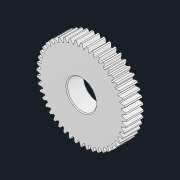
# Autodesk Inventor part: unit-planet_gear
Saved by Autodesk Inventor 2021 (Build 250183000, 183)
## iProperties
Created: 2021-07-12
Part Number: unit-planet_gear
Material: ABS プラスチック
Document SubType Name: Modeling
Designer: yuta0
Density: 1.06 g/cm^3
Appearance: 滑らか - 白
購入先: 印刷
在庫数: 0.0
Author: yuta0
Autodesk Inventor part; units mm, degrees
ref_plane "YZ Plane" through (0, 0, 0) normal (1, 0, 0) x (0, 1, 0)
ref_plane "XZ Plane" through (0, 0, 0) normal (0, 1, 0) x (-1, 0, 0)
ref_plane "XY Plane" through (0, 0, 0) normal (0, 0, 1) x (1, 0, 0)
sketch "スケッチ1" plane through (0, 0, 0) normal (0, 0, 1) x (1, 0, 0)
  arc A0 (-3.6816, 24.8194) -> (-4.0891, 22.473) centre (7.7013, 21.6341) ccw
  arc A1 (-4.0891, 22.473) -> (-4.8222, 22.3272) centre (0, 0) ccw
  arc A2 (-4.8222, 22.3272) -> (-6.0966, 24.3391) centre (-15.394, 17.0401) ccw
  arc A3 (-6.0966, 24.3391) -> (-6.8897, 24.1266) centre (0, 0) ccw
  arc A4 (-6.8897, 24.1266) -> (-6.9874, 21.747) centre (4.8116, 22.4542) ccw
  arc A5 (-6.9874, 21.747) -> (-7.6952, 21.5067) centre (0, 0) ccw
  arc A6 (-7.6952, 21.5067) -> (-9.2213, 23.3351) centre (-17.4865, 14.885) ccw
  arc A7 (-9.2213, 23.3351) -> (-9.9799, 23.0209) centre (0, 0) ccw
  arc A8 (-9.9799, 23.0209) -> (-9.7662, 20.6489) centre (1.8395, 22.8902) ccw
  arc A9 (-9.7662, 20.6489) -> (-10.4366, 20.3183) centre (0, 0) ccw
  arc A10 (-10.4366, 20.3183) -> (-12.1883, 21.9318) centre (-19.2798, 12.4752) ccw
  arc A11 (-12.1883, 21.9318) -> (-12.8994, 21.5213) centre (0, 0) ccw
  arc A12 (-12.8994, 21.5213) -> (-12.3779, 19.1975) centre (-1.164, 22.9344) ccw
  arc A13 (-12.3779, 19.1975) -> (-12.9994, 18.7822) centre (0, 0) ccw
  arc A14 (-12.9994, 18.7822) -> (-14.9467, 20.1533) centre (-20.7432, 9.852) ccw
  arc A15 (-14.9467, 20.1533) -> (-15.5981, 19.6535) centre (0, 0) ccw
  arc A16 (-15.5981, 19.6535) -> (-14.7778, 17.4176) centre (-4.1476, 22.5863) ccw
  arc A17 (-14.7778, 17.4176) -> (-15.3397, 16.9248) centre (0, 0) ccw
  arc A18 (-15.3397, 16.9248) -> (-17.4494, 18.0299) centre (-21.8517, 7.0602) ccw
  arc A19 (-17.4494, 18.0299) -> (-18.0299, 17.4494) centre (0, 0) ccw
  arc A20 (-18.0299, 17.4494) -> (-16.9248, 15.3397) centre (-7.0602, 21.8517) ccw
  arc A21 (-16.9248, 15.3397) -> (-17.4176, 14.7778) centre (0, 0) ccw
  arc A22 (-17.4176, 14.7778) -> (-19.6535, 15.5981) centre (-22.5863, 4.1476) ccw
  arc A23 (-19.6535, 15.5981) -> (-20.1533, 14.9467) centre (0, 0) ccw
  arc A24 (-20.1533, 14.9467) -> (-18.7822, 12.9994) centre (-9.852, 20.7432) ccw
  arc A25 (-18.7822, 12.9994) -> (-19.1975, 12.3779) centre (0, 0) ccw
  arc A26 (-19.1975, 12.3779) -> (-21.5213, 12.8994) centre (-22.9344, 1.164) ccw
  arc A27 (-21.5213, 12.8994) -> (-21.9318, 12.1883) centre (0, 0) ccw
  arc A28 (-21.9318, 12.1883) -> (-20.3183, 10.4366) centre (-12.4752, 19.2798) ccw
  arc A29 (-20.3183, 10.4366) -> (-20.6489, 9.7662) centre (0, 0) ccw
  arc A30 (-20.6489, 9.7662) -> (-23.0209, 9.9799) centre (-22.8902, -1.8395) ccw
  arc A31 (-23.0209, 9.9799) -> (-23.3351, 9.2213) centre (0, 0) ccw
  arc A32 (-23.3351, 9.2213) -> (-21.5067, 7.6952) centre (-14.885, 17.4865) ccw
  arc A33 (-21.5067, 7.6952) -> (-21.747, 6.9874) centre (0, 0) ccw
  arc A34 (-21.747, 6.9874) -> (-24.1266, 6.8897) centre (-22.4542, -4.8116) ccw
  arc A35 (-24.1266, 6.8897) -> (-24.3391, 6.0966) centre (0, 0) ccw
  arc A36 (-24.3391, 6.0966) -> (-22.3272, 4.8222) centre (-17.0401, 15.394) ccw
  arc A37 (-22.3272, 4.8222) -> (-22.473, 4.0891) centre (0, 0) ccw
  arc A38 (-22.473, 4.0891) -> (-24.8194, 3.6816) centre (-21.6341, -7.7013) ccw
  arc A39 (-24.8194, 3.6816) -> (-24.9266, 2.8676) centre (0, 0) ccw
  arc A40 (-24.9266, 2.8676) -> (-22.7656, 1.8667) centre (-18.9037, 13.0382) ccw
  arc A41 (-22.7656, 1.8667) -> (-22.8145, 1.1208) centre (0, 0) ccw
  arc A42 (-22.8145, 1.1208) -> (-25.0876, 0.4105) centre (-20.4438, -10.4592) ccw
  arc A43 (-25.0876, 0.4105) -> (-25.0876, -0.4105) centre (0, 0) ccw
  arc A44 (-25.0876, -0.4105) -> (-22.8145, -1.1208) centre (-20.4438, 10.4592) ccw
  arc A45 (-22.8145, -1.1208) -> (-22.7656, -1.8667) centre (0, 0) ccw
  arc A46 (-22.7656, -1.8667) -> (-24.9266, -2.8676) centre (-18.9037, -13.0382) ccw
  arc A47 (-24.9266, -2.8676) -> (-24.8194, -3.6816) centre (0, 0) ccw
  arc A48 (-24.8194, -3.6816) -> (-22.473, -4.0891) centre (-21.6341, 7.7013) ccw
  arc A49 (-22.473, -4.0891) -> (-22.3272, -4.8222) centre (0, 0) ccw
  arc A50 (-22.3272, -4.8222) -> (-24.3391, -6.0966) centre (-17.0401, -15.394) ccw
  arc A51 (-24.3391, -6.0966) -> (-24.1266, -6.8897) centre (0, 0) ccw
  arc A52 (-24.1266, -6.8897) -> (-21.747, -6.9874) centre (-22.4542, 4.8116) ccw
  arc A53 (-21.747, -6.9874) -> (-21.5067, -7.6952) centre (0, 0) ccw
  arc A54 (-21.5067, -7.6952) -> (-23.3351, -9.2213) centre (-14.885, -17.4865) ccw
  arc A55 (-23.3351, -9.2213) -> (-23.0209, -9.9799) centre (0, 0) ccw
  arc A56 (-23.0209, -9.9799) -> (-20.6489, -9.7662) centre (-22.8902, 1.8395) ccw
  arc A57 (-20.6489, -9.7662) -> (-20.3183, -10.4366) centre (0, 0) ccw
  arc A58 (-20.3183, -10.4366) -> (-21.9318, -12.1883) centre (-12.4752, -19.2798) ccw
  arc A59 (-21.9318, -12.1883) -> (-21.5213, -12.8994) centre (0, 0) ccw
  arc A60 (-21.5213, -12.8994) -> (-19.1975, -12.3779) centre (-22.9344, -1.164) ccw
  arc A61 (-19.1975, -12.3779) -> (-18.7822, -12.9994) centre (0, 0) ccw
  arc A62 (-18.7822, -12.9994) -> (-20.1533, -14.9467) centre (-9.852, -20.7432) ccw
  arc A63 (-20.1533, -14.9467) -> (-19.6535, -15.5981) centre (0, 0) ccw
  arc A64 (-19.6535, -15.5981) -> (-17.4176, -14.7778) centre (-22.5863, -4.1476) ccw
  arc A65 (-17.4176, -14.7778) -> (-16.9248, -15.3397) centre (0, 0) ccw
  arc A66 (-16.9248, -15.3397) -> (-18.0299, -17.4494) centre (-7.0602, -21.8517) ccw
  arc A67 (-18.0299, -17.4494) -> (-17.4494, -18.0299) centre (0, 0) ccw
  arc A68 (-17.4494, -18.0299) -> (-15.3397, -16.9248) centre (-21.8517, -7.0602) ccw
  arc A69 (-15.3397, -16.9248) -> (-14.7778, -17.4176) centre (0, 0) ccw
  arc A70 (-14.7778, -17.4176) -> (-15.5981, -19.6535) centre (-4.1476, -22.5863) ccw
  arc A71 (-15.5981, -19.6535) -> (-14.9467, -20.1533) centre (0, 0) ccw
  arc A72 (-14.9467, -20.1533) -> (-12.9994, -18.7822) centre (-20.7432, -9.852) ccw
  arc A73 (-12.9994, -18.7822) -> (-12.3779, -19.1975) centre (0, 0) ccw
  arc A74 (-12.3779, -19.1975) -> (-12.8994, -21.5213) centre (-1.164, -22.9344) ccw
  arc A75 (-12.8994, -21.5213) -> (-12.1883, -21.9318) centre (0, 0) ccw
  arc A76 (-12.1883, -21.9318) -> (-10.4366, -20.3183) centre (-19.2798, -12.4752) ccw
  arc A77 (-10.4366, -20.3183) -> (-9.7662, -20.6489) centre (0, 0) ccw
  arc A78 (-9.7662, -20.6489) -> (-9.9799, -23.0209) centre (1.8395, -22.8902) ccw
  arc A79 (-9.9799, -23.0209) -> (-9.2213, -23.3351) centre (0, 0) ccw
  arc A80 (-9.2213, -23.3351) -> (-7.6952, -21.5067) centre (-17.4865, -14.885) ccw
  arc A81 (-7.6952, -21.5067) -> (-6.9874, -21.747) centre (0, 0) ccw
  arc A82 (-6.9874, -21.747) -> (-6.8897, -24.1266) centre (4.8116, -22.4542) ccw
  arc A83 (-6.8897, -24.1266) -> (-6.0966, -24.3391) centre (0, 0) ccw
  arc A84 (-6.0966, -24.3391) -> (-4.8222, -22.3272) centre (-15.394, -17.0401) ccw
  arc A85 (-4.8222, -22.3272) -> (-4.0891, -22.473) centre (0, 0) ccw
  arc A86 (-4.0891, -22.473) -> (-3.6816, -24.8194) centre (7.7013, -21.6341) ccw
  arc A87 (-3.6816, -24.8194) -> (-2.8676, -24.9266) centre (0, 0) ccw
  arc A88 (-2.8676, -24.9266) -> (-1.8667, -22.7656) centre (-13.0382, -18.9037) ccw
  arc A89 (-1.8667, -22.7656) -> (-1.1208, -22.8145) centre (0, 0) ccw
  arc A90 (-1.1208, -22.8145) -> (-0.4105, -25.0876) centre (10.4592, -20.4438) ccw
  arc A91 (-0.4105, -25.0876) -> (0.4105, -25.0876) centre (0, 0) ccw
  arc A92 (0.4105, -25.0876) -> (1.1208, -22.8145) centre (-10.4592, -20.4438) ccw
  arc A93 (1.1208, -22.8145) -> (1.8667, -22.7656) centre (0, 0) ccw
  arc A94 (1.8667, -22.7656) -> (2.8676, -24.9266) centre (13.0382, -18.9037) ccw
  arc A95 (2.8676, -24.9266) -> (3.6816, -24.8194) centre (0, 0) ccw
  arc A96 (3.6816, -24.8194) -> (4.0891, -22.473) centre (-7.7013, -21.6341) ccw
  arc A97 (4.0891, -22.473) -> (4.8222, -22.3272) centre (0, 0) ccw
  arc A98 (4.8222, -22.3272) -> (6.0966, -24.3391) centre (15.394, -17.0401) ccw
  arc A99 (6.0966, -24.3391) -> (6.8897, -24.1266) centre (0, 0) ccw
  arc A100 (6.8897, -24.1266) -> (6.9874, -21.747) centre (-4.8116, -22.4542) ccw
  arc A101 (6.9874, -21.747) -> (7.6952, -21.5067) centre (0, 0) ccw
  arc A102 (7.6952, -21.5067) -> (9.2213, -23.3351) centre (17.4865, -14.885) ccw
  arc A103 (9.2213, -23.3351) -> (9.9799, -23.0209) centre (0, 0) ccw
  arc A104 (9.9799, -23.0209) -> (9.7662, -20.6489) centre (-1.8395, -22.8902) ccw
  arc A105 (9.7662, -20.6489) -> (10.4366, -20.3183) centre (0, 0) ccw
  arc A106 (10.4366, -20.3183) -> (12.1883, -21.9318) centre (19.2798, -12.4752) ccw
  arc A107 (12.1883, -21.9318) -> (12.8994, -21.5213) centre (0, 0) ccw
  arc A108 (12.8994, -21.5213) -> (12.3779, -19.1975) centre (1.164, -22.9344) ccw
  arc A109 (12.3779, -19.1975) -> (12.9994, -18.7822) centre (0, 0) ccw
  arc A110 (12.9994, -18.7822) -> (14.9467, -20.1533) centre (20.7432, -9.852) ccw
  arc A111 (14.9467, -20.1533) -> (15.5981, -19.6535) centre (0, 0) ccw
  arc A112 (15.5981, -19.6535) -> (14.7778, -17.4176) centre (4.1476, -22.5863) ccw
  arc A113 (14.7778, -17.4176) -> (15.3397, -16.9248) centre (0, 0) ccw
  arc A114 (15.3397, -16.9248) -> (17.4494, -18.0299) centre (21.8517, -7.0602) ccw
  arc A115 (17.4494, -18.0299) -> (18.0299, -17.4494) centre (0, 0) ccw
  arc A116 (18.0299, -17.4494) -> (16.9248, -15.3397) centre (7.0602, -21.8517) ccw
  arc A117 (16.9248, -15.3397) -> (17.4176, -14.7778) centre (0, 0) ccw
  arc A118 (17.4176, -14.7778) -> (19.6535, -15.5981) centre (22.5863, -4.1476) ccw
  arc A119 (19.6535, -15.5981) -> (20.1533, -14.9467) centre (0, 0) ccw
  arc A120 (20.1533, -14.9467) -> (18.7822, -12.9994) centre (9.852, -20.7432) ccw
  arc A121 (18.7822, -12.9994) -> (19.1975, -12.3779) centre (0, 0) ccw
  arc A122 (19.1975, -12.3779) -> (21.5213, -12.8994) centre (22.9344, -1.164) ccw
  arc A123 (21.5213, -12.8994) -> (21.9318, -12.1883) centre (0, 0) ccw
  arc A124 (21.9318, -12.1883) -> (20.3183, -10.4366) centre (12.4752, -19.2798) ccw
  arc A125 (20.3183, -10.4366) -> (20.6489, -9.7662) centre (0, 0) ccw
  arc A126 (20.6489, -9.7662) -> (23.0209, -9.9799) centre (22.8902, 1.8395) ccw
  arc A127 (23.0209, -9.9799) -> (23.3351, -9.2213) centre (0, 0) ccw
  arc A128 (23.3351, -9.2213) -> (21.5067, -7.6952) centre (14.885, -17.4865) ccw
  arc A129 (21.5067, -7.6952) -> (21.747, -6.9874) centre (0, 0) ccw
  arc A130 (21.747, -6.9874) -> (24.1266, -6.8897) centre (22.4542, 4.8116) ccw
  arc A131 (24.1266, -6.8897) -> (24.3391, -6.0966) centre (0, 0) ccw
  arc A132 (24.3391, -6.0966) -> (22.3272, -4.8222) centre (17.0401, -15.394) ccw
  arc A133 (22.3272, -4.8222) -> (22.473, -4.0891) centre (0, 0) ccw
  arc A134 (22.473, -4.0891) -> (24.8194, -3.6816) centre (21.6341, 7.7013) ccw
  arc A135 (24.8194, -3.6816) -> (24.9266, -2.8676) centre (0, 0) ccw
  arc A136 (24.9266, -2.8676) -> (22.7656, -1.8667) centre (18.9037, -13.0382) ccw
  arc A137 (22.7656, -1.8667) -> (22.8145, -1.1208) centre (0, 0) ccw
  arc A138 (22.8145, -1.1208) -> (25.0876, -0.4105) centre (20.4438, 10.4592) ccw
  arc A139 (25.0876, -0.4105) -> (25.0876, 0.4105) centre (0, 0) ccw
  arc A140 (25.0876, 0.4105) -> (22.8145, 1.1208) centre (20.4438, -10.4592) ccw
  arc A141 (22.8145, 1.1208) -> (22.7656, 1.8667) centre (0, 0) ccw
  arc A142 (22.7656, 1.8667) -> (24.9266, 2.8676) centre (18.9037, 13.0382) ccw
  arc A143 (24.9266, 2.8676) -> (24.8194, 3.6816) centre (0, 0) ccw
  arc A144 (24.8194, 3.6816) -> (22.473, 4.0891) centre (21.6341, -7.7013) ccw
  arc A145 (22.473, 4.0891) -> (22.3272, 4.8222) centre (0, 0) ccw
  arc A146 (22.3272, 4.8222) -> (24.3391, 6.0966) centre (17.0401, 15.394) ccw
  arc A147 (24.3391, 6.0966) -> (24.1266, 6.8897) centre (0, 0) ccw
  arc A148 (24.1266, 6.8897) -> (21.747, 6.9874) centre (22.4542, -4.8116) ccw
  arc A149 (21.747, 6.9874) -> (21.5067, 7.6952) centre (0, 0) ccw
  arc A150 (21.5067, 7.6952) -> (23.3351, 9.2213) centre (14.885, 17.4865) ccw
  arc A151 (23.3351, 9.2213) -> (23.0209, 9.9799) centre (0, 0) ccw
  arc A152 (23.0209, 9.9799) -> (20.6489, 9.7662) centre (22.8902, -1.8395) ccw
  arc A153 (20.6489, 9.7662) -> (20.3183, 10.4366) centre (0, 0) ccw
  arc A154 (20.3183, 10.4366) -> (21.9318, 12.1883) centre (12.4752, 19.2798) ccw
  arc A155 (21.9318, 12.1883) -> (21.5213, 12.8994) centre (0, 0) ccw
  arc A156 (21.5213, 12.8994) -> (19.1975, 12.3779) centre (22.9344, 1.164) ccw
  arc A157 (19.1975, 12.3779) -> (18.7822, 12.9994) centre (0, 0) ccw
  arc A158 (18.7822, 12.9994) -> (20.1533, 14.9467) centre (9.852, 20.7432) ccw
  arc A159 (20.1533, 14.9467) -> (19.6535, 15.5981) centre (0, 0) ccw
  arc A160 (19.6535, 15.5981) -> (17.4176, 14.7778) centre (22.5863, 4.1476) ccw
  arc A161 (17.4176, 14.7778) -> (16.9248, 15.3397) centre (0, 0) ccw
  arc A162 (16.9248, 15.3397) -> (18.0299, 17.4494) centre (7.0602, 21.8517) ccw
  arc A163 (18.0299, 17.4494) -> (17.4494, 18.0299) centre (0, 0) ccw
  arc A164 (17.4494, 18.0299) -> (15.3397, 16.9248) centre (21.8517, 7.0602) ccw
  arc A165 (15.3397, 16.9248) -> (14.7778, 17.4176) centre (0, 0) ccw
  arc A166 (14.7778, 17.4176) -> (15.5981, 19.6535) centre (4.1476, 22.5863) ccw
  arc A167 (15.5981, 19.6535) -> (14.9467, 20.1533) centre (0, 0) ccw
  arc A168 (14.9467, 20.1533) -> (12.9994, 18.7822) centre (20.7432, 9.852) ccw
  arc A169 (12.9994, 18.7822) -> (12.3779, 19.1975) centre (0, 0) ccw
  arc A170 (12.3779, 19.1975) -> (12.8994, 21.5213) centre (1.164, 22.9344) ccw
  arc A171 (12.8994, 21.5213) -> (12.1883, 21.9318) centre (0, 0) ccw
  arc A172 (12.1883, 21.9318) -> (10.4366, 20.3183) centre (19.2798, 12.4752) ccw
  arc A173 (10.4366, 20.3183) -> (9.7662, 20.6489) centre (0, 0) ccw
  arc A174 (9.7662, 20.6489) -> (9.9799, 23.0209) centre (-1.8395, 22.8902) ccw
  arc A175 (9.9799, 23.0209) -> (9.2213, 23.3351) centre (0, 0) ccw
  arc A176 (9.2213, 23.3351) -> (7.6952, 21.5067) centre (17.4865, 14.885) ccw
  arc A177 (7.6952, 21.5067) -> (6.9874, 21.747) centre (0, 0) ccw
  arc A178 (6.9874, 21.747) -> (6.8897, 24.1266) centre (-4.8116, 22.4542) ccw
  arc A179 (6.8897, 24.1266) -> (6.0966, 24.3391) centre (0, 0) ccw
  arc A180 (6.0966, 24.3391) -> (4.8222, 22.3272) centre (15.394, 17.0401) ccw
  arc A181 (4.8222, 22.3272) -> (4.0891, 22.473) centre (0, 0) ccw
  arc A182 (4.0891, 22.473) -> (3.6816, 24.8194) centre (-7.7013, 21.6341) ccw
  arc A183 (3.6816, 24.8194) -> (2.8676, 24.9266) centre (0, 0) ccw
  arc A184 (2.8676, 24.9266) -> (1.8667, 22.7656) centre (13.0382, 18.9037) ccw
  arc A185 (1.8667, 22.7656) -> (1.1208, 22.8145) centre (0, 0) ccw
  arc A186 (1.1208, 22.8145) -> (0.4105, 25.0876) centre (-10.4592, 20.4438) ccw
  arc A187 (0.4105, 25.0876) -> (-0.4105, 25.0876) centre (0, 0) ccw
  arc A188 (-0.4105, 25.0876) -> (-1.1208, 22.8145) centre (10.4592, 20.4438) ccw
  arc A189 (-1.1208, 22.8145) -> (-1.8667, 22.7656) centre (0, 0) ccw
  arc A190 (-1.8667, 22.7656) -> (-2.8676, 24.9266) centre (-13.0382, 18.9037) ccw
  arc A191 (-2.8676, 24.9266) -> (-3.6816, 24.8194) centre (0, 0) ccw
  constraints: 384 point on circle, 192 centre point, 578 other
extrude "押し出し1" add sketch "スケッチ1" along normal mid plane 9.8
sketch "スケッチ2" plane through (0, 0, 4.9) normal (0, 0, 1) x (1, 0, 0)
  circle A0 centre (0, 0) radius 8.1
  dimension "d2" = 16.2
  constraints: 1 centre point, 1 coincident
  measures "d2" diameter of A0
extrude "押し出し2" cut sketch "スケッチ2" against normal through all
chamfer "面取り1" distance 0.5 angle 45 2 edges at (-8.1, 0, 4.9) (-8.1, 0, -4.9)
